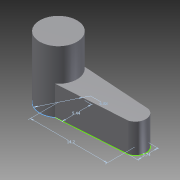
# Autodesk Inventor part: Robot_ARM_Pivot
Saved by Autodesk Inventor 2011 SP2 (Build 150309200, 309)
## iProperties
Created: 2015-11-08
Part Number: Robot_ARM_Pivot
Document SubType Name: Modeling
Designer: Ernest
Density: 1 g/cm^3
Author: Ernest
Autodesk Inventor part; units mm, degrees
ref_plane "YZ Plane" through (0, 0, 0) normal (1, 0, 0) x (0, 1, 0)
ref_plane "XZ Plane" through (0, 0, 0) normal (0, 1, 0) x (-1, 0, 0)
ref_plane "XY Plane" through (0, 0, 0) normal (0, 0, 1) x (1, 0, 0)
sketch "Sketch1" plane through (0, 0, 0) normal (0, 0, 1) x (1, 0, 0)
  circle A0 centre (0, 0) radius 3.44
  line L0 (2.106, 2.72) -> (2.106, -2.72) construction
  line L1 (14.7702, 1.87) -> (14.7702, -1.87) construction
  line L2 (2.106, 2.72) -> (14.7702, 1.87)
  line L3 (14.7702, -1.87) -> (2.106, -2.72)
  arc A1 (14.7702, -1.87) -> (14.7702, 1.87) centre (14.2, 0) ccw
  dimension "d0" = 6.88
  dimension "d2" = 14.2
  dimension "d3" = 5.44
  dimension "d4" = 3.74
  constraints: 8 end point, 5 point on circle, 2 centre point, 1 coincident, 1 parallel, 1 vertical
  measures "d0" diameter of A0
  measures "d2" distance of A1.centre point (0, 0)
  measures "d3" distance of L0.start L0.end
  measures "d4" distance of L1.start L1.end
extrude "Extrusion1" add sketch "Sketch1" along normal blind 5.384 contours A0 L2 A1 L3
extrude "Extrusion2" add sketch "Sketch1" along normal blind 11.384 contours A0
body "Solid1"
